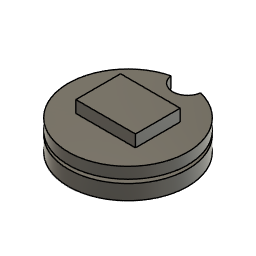
locking ring construction (Autodesk Fusion 360 design; units mm, degrees)
Autodesk Fusion 360 part; units mm, degrees
note: some values were not read from the file. Set by a fixed rule: which sketch regions a step uses.
sketch "Sketch1" plane through (0, 0, 0) normal (0, 1, 0) x (1, 0, 0)
  circle A0 centre (0, 0) radius 25.4
  dimension "d1" = 50.8
  constraint coincident A0.centre origin
  measures "d1" diameter of A0
extrude "Extrude1" add sketch "Sketch1" along normal blind 12.7
sketch "Sketch2" plane through (0, 12.7, 0) normal (0, 1, 0) x (-1, 0, 0)
  circle A0 centre (0, 0) radius 25.4
  circle A1 centre (0, -25.4) radius 6.35
  dimension "d4" = 12.7
  constraint coincident A0 A1.centre
  constraint vertical A0.centre A1.centre
  measures "d4" diameter of A1
extrude "Extrude2" cut sketch "Sketch2" against normal blind 6.35 contours A0 A1 | A0 A1 picked at (-1.9477, -23.4128) picked at (2.1308, -27.1585)
sketch "Sketch3" plane through (0, 12.7, 0) normal (0, 1, 0) x (-1, 0, 0)
  arc A0 (6.3002, -24.6062) -> (-6.3002, -24.6062) centre (0, -25.4) ccw
  arc A1 (6.3002, -24.6063) -> (-6.3002, -24.6062) centre (0, 0) ccw
  circle A2 centre (0, -10.795) radius 4.7625
  circle A3 centre (0, -10.795) radius 2.5527
  dimension "d7" = 9.525
  dimension "d8" = 10.795
  dimension "d9" = 5.1054
  constraint vertical A1.centre A2.centre
  constraint concentric A2 A3
  measures "d7" diameter of A2
  measures "d8" distance of A1.centre A2.centre
  measures "d9" diameter of A3
sketch "Sketch4" plane through (0, 0, 0) normal (1, 0, 0) x (0, 0, -1)
  line L0 (25.4, 0) -> (25.4, 6.35)
  line L1 (-25.4, 12.7) -> (-25.4, 0)
  line L2 (19.05, 6.35) -> (24.6062, 6.35)
  line L3 (25.4, 6.35) -> (22.225, 6.35)
  line L4 (22.225, 7.9375) -> (25.4, 7.9375)
  line L5 (25.4, 7.9375) -> (25.4, 6.35)
  line L6 (22.225, 7.9375) -> (22.225, 6.35)
  dimension "d12" = 3.175
  dimension "d13" = 1.5875
  constraint coincident L0.end L3.start
  constraint coincident L2 L3.end
  constraint perpendicular L0 L3
  constraint perpendicular L0 L4
  constraint perpendicular L3 L5
  constraint perpendicular L2 L6
  measures "d12" distance of L0.end L3.end
  measures "d13" distance of L4.end L0.end
revolve "Revolve1" cut sketch "Sketch4" angle 360 about axis through (0, 1.75, 0) along (0, 1, 0)
sketch "Sketch5" plane through (0, 12.7, 0) normal (0, 1, 0) x (-1, 0, 0)
  arc A0 (6.3002, -24.6062) -> (-6.3002, -24.6062) centre (0, -25.4) ccw
  arc A1 (6.3002, -24.6063) -> (-6.3002, -24.6062) centre (0, 0) ccw
  line L0 (0, -19.05) -> (0, 0) construction
  line L1 (0, 0) -> (0, 19.05) construction
  circle A2 centre (0, 25.4) radius 6.35
  arc A3 (5.1095, -21.6297) -> (-5.1095, -21.6297) centre (0, 0) ccw
  line L2 (-12.7, 9.525) -> (12.7, 9.525)
  line L3 (12.7, 9.525) -> (12.7, -9.525)
  line L4 (12.7, -9.525) -> (-12.7, -9.525)
  line L5 (-12.7, -9.525) -> (-12.7, 9.525)
  line L6 (-12.7, 9.525) -> (12.7, -9.525) construction
  line L7 (12.7, 9.525) -> (-12.7, -9.525) construction
  circle A4 centre (0, 0) radius 15.875
  dimension "d15" = 25.4
  dimension "d16" = 19.05
  dimension "d17" = 31.75
  constraint midpoint A0 L0.start
  constraint coincident A1.centre L0.end
  constraint parallel L0 L1
  constraint equal L0 L1
  constraint coincident L1.end A2
  constraint equal A0 A2
  constraint vertical A1.centre A2.centre
  constraint horizontal L2
  constraint perpendicular L2 L3
  constraint parallel L2 L4
  constraint parallel L3 L5
  constraint coincident L6 A1.centre
  constraint coincident L7 A1.centre
  constraint concentric A3 A4
  measures "d15" distance of L3.end L4.end
  measures "d16" distance of L2.end L3.end
  measures "d17" diameter of A4
extrude "Extrude4" add sketch "Sketch5" along normal blind 5.08 contours L2 L3 L4 L5
equation "d17 = d15 + 0.25 in"
